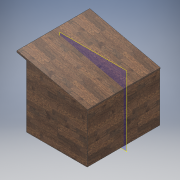
# Autodesk Inventor part: Top
Saved by Autodesk Inventor 2017 (Build 210142000, 142)
## iProperties
Created: 2016-09-09
Part Number: Top
Material: Generic
Document SubType Name: Modeling
Designer: s.ethan.wierenga
Density: 1 g/cm^3
Appearance: White Ash - Java
Author: s.ethan.wierenga
Autodesk Inventor part; units mm, degrees
ref_plane "YZ Plane" through (0, 0, 0) normal (1, 0, 0) x (0, 1, 0)
ref_plane "XZ Plane" through (0, 0, 0) normal (0, 1, 0) x (-1, 0, 0)
ref_plane "XY Plane" through (0, 0, 0) normal (0, 0, 1) x (1, 0, 0)
sketch "Sketch1" plane through (0, 0, 0) normal (0, 1, 0) x (-1, 0, 0)
  line L0 (0, 0) -> (-762, 0)
  line L1 (-762, 0) -> (-762, -914.4)
  line L2 (-762, -914.4) -> (0, -914.4)
  line L3 (0, -914.4) -> (0, 0)
  dimension "d0" = 762
  dimension "d1" = 914.4
  constraints: 8 end point, 2 parallel, 1 horizontal, 1 perpendicular
  measures "d0" distance of L2.end L1.end
  measures "d1" distance of L1.end L0.end
extrude "Extrusion1" add sketch "Sketch1" along normal blind 19.05
sketch "Sketch5" plane through (762, 0, -914.4) normal (0, 0, -1) x (-1, 0, 0)
  line L0 (0, 0) -> (0, 19.05) projected
  line L1 (0, 0) -> (762, 0) projected
  line L2 (762, 0) -> (762, 19.05) projected
  line L3 (762, 628.65) -> (762, 781.05)
  line L4 (762, 781.05) -> (0, 609.6)
  line L5 (0, 609.6) -> (762, 609.6) construction
  line L6 (762, 19.05) -> (762, 628.65) construction
  line L7 (762, 781.05) -> (757.8183, 799.6354)
  line L8 (757.8183, 799.6354) -> (-4.1817, 628.1854)
  line L9 (0, 609.6) -> (84.6693, 628.65) projected
  line L10 (-4.1817, 628.1854) -> (0, 609.6)
  line L11 (0, 19.05) -> (762, 19.05) projected
  dimension "d22" = 152.4
  dimension "d23" = 12.68
  dimension "d25" = 19.05
  dimension "d26" = 90
  dimension "d28" = 90
  dimension "d29" = 90
  constraints: 12 end point, 1 perpendicular, 1 point on line, 1 vertical
  measures "d22" distance of L3.start L3.end
  measures "d23" angle of L5 L4
  measures "d25" distance of L3.end L7.end
  measures "d26" angle of L7 L4
  measures "d28" angle of L4 L10
  measures "d29" angle of L8 L10
extrude "Extrusion5" add sketch "Sketch5" against normal up to surface (914.4 mm away) contours L4 L10 L8 L7
sketch "Sketch7" plane through (0, 19.05, 0) normal (0, 1, 0) x (1, 0, 0)
  line L0 (0, 0) -> (762, 0) projected
  line L1 (0, 914.4) -> (0, 0) projected
  line L2 (762, 914.4) -> (0, 914.4) projected
  line L3 (762, 0) -> (762, 914.4) projected
  line L4 (762, 0) -> (762, 914.4) projected
  line L5 (0, 914.4) -> (0, 0) projected
  line L6 (762, 914.4) -> (0, 914.4)
  line L7 (0, 914.4) -> (0, 895.35)
  line L8 (0, 895.35) -> (742.95, 895.35)
  line L9 (762, 895.35) -> (762, 914.4)
  line L10 (762, 914.4) -> (742.95, 914.4)
  line L11 (742.95, 895.35) -> (742.95, 457.2)
  line L12 (742.95, 457.2) -> (762, 457.2)
  line L13 (762, 457.2) -> (762, 914.4)
  dimension "d38" = 19.05
  dimension "d39" = 19.05
  dimension "d40" = 457.2
  constraints: 16 end point, 4 parallel, 2 horizontal, 2 perpendicular, 1 point on line
  measures "d38" distance of L7.end L6.end
  measures "d39" distance of L12.end L11.end
  measures "d40" distance of L11.end L10.end
extrude "Extrusion7" add sketch "Sketch7" along normal blind 609.6 contours L1 L2 L3 L12 L11 L8
sketch "Sketch8" plane through (762, 0, -914.4) normal (0, 0, -1) x (-1, 0, 0)
  line L0 (0, 0) -> (762, 0) projected
  line L1 (762, 0) -> (762, 628.65) projected
  line L2 (84.6667, 628.65) -> (762, 628.65) projected
  line L3 (84.6667, 628.65) -> (762, 781.05) projected
  line L4 (762, 781.05) -> (757.8183, 799.6354) projected
  line L5 (757.8183, 799.6354) -> (-4.1817, 628.1854) projected
  line L6 (-4.1817, 628.1854) -> (0, 609.6) projected
  line L7 (0, 0) -> (0, 609.6) projected
  line L8 (762, 628.65) -> (762, 781.05)
  line L9 (84.6667, 628.65) -> (762, 781.05) projected
  line L10 (762, 781.05) -> (84.6667, 628.65)
  line L11 (84.6667, 628.65) -> (762, 628.65)
  constraints: 6 end point, 1 collinear, 1 perpendicular, 1 vertical
extrude "Extrusion8" add sketch "Sketch8" against normal blind 19.05 contours L2 L3 L8
ref_plane "Work Plane2" through (762, 0, -457.2) normal (0, 0, -1) x (-1, 0, 0)
mirror "Mirror1" about plane through (762, 0, -457.2) normal (0, 0, -1) of "Extrusion7"
sketch "Sketch9" plane through (0, 0, 0) normal (0, 0, 1) x (1, 0, 0)
  line L0 (766.1817, 628.1854) -> (762, 609.6) projected
  line L1 (4.1817, 799.6354) -> (766.1817, 628.1854) projected
  line L2 (0, 781.05) -> (4.1817, 799.6354) projected
  line L3 (677.3333, 628.65) -> (0, 781.05) projected
  line L4 (677.3333, 628.65) -> (0, 628.65) projected
  line L5 (0, 0) -> (0, 628.65) projected
  line L6 (0, 0) -> (762, 0) projected
  line L7 (762, 0) -> (762, 609.6) projected
  line L8 (0, 19.05) -> (0, 781.05) projected
  line L9 (0, 628.65) -> (0, 781.05)
  line L10 (0, 781.05) -> (677.3333, 628.65)
  line L11 (0, 781.05) -> (742.95, 613.8863) projected
  line L12 (0, 628.65) -> (677.3333, 628.65)
  constraints: 6 end point, 2 collinear, 1 perpendicular
extrude "Extrusion9" add sketch "Sketch9" against normal blind 19.05 contours L3 L4 L8
sketch "Sketch12" plane through (742.95, 19.05, -895.35) normal (-1, 0, 0) x (0, 0, 1)
  line L0 (0, 594.8363) -> (876.3, 594.8363) projected
  line L1 (0, 0) -> (0, 594.8363) projected
  line L2 (876.3, 0) -> (0, 0) projected
  line L3 (876.3, 0) -> (876.3, 594.8363) projected
  line L4 (0, 0) -> (0, 594.8363) projected
  line L5 (876.3, 0) -> (876.3, 762) projected
  line L6 (0, 442.4363) -> (876.3, 442.4363)
  line L7 (876.3, 442.4363) -> (876.3, 423.3862)
  line L8 (876.3, 423.3862) -> (0, 423.3862)
  line L9 (0, 423.3862) -> (0, 442.4363)
  point P0 (895.35, -19.05)
  dimension "d57" = 19.05
  dimension "d58" = 152.4
  constraints: 8 end point, 2 parallel, 2 point on line, 1 horizontal, 1 perpendicular
  measures "d57" distance of L6.end L7.end
  measures "d58" distance between parallel lines of L0 L6
extrude "Extrusion10" add sketch "Sketch12" along normal up to surface (742.95 mm away) contours L6 L3 L8 L1
sketch "Sketch13" plane through (742.95, 461.4863, -19.05) normal (0, 1, 0) x (1, 0, 0)
  line L0 (-742.95, 0) -> (-742.95, 876.3) projected
  line L1 (0, 876.3) -> (-742.95, 876.3) projected
  line L2 (0, 0) -> (0, 876.3) projected
  line L3 (-742.95, 0) -> (0, 0) projected
  line L4 (0, 0) -> (0, 876.3) projected
  line L5 (-742.95, 876.3) -> (-742.95, 0) projected
  line L6 (0, 438.15) -> (-742.95, 438.15)
  line L7 (-742.95, 438.15) -> (-742.95, 419.1)
  line L8 (-742.95, 419.1) -> (0, 419.1)
  line L9 (0, 419.1) -> (0, 438.15)
  point P0 (-742.95, -19.05)
  dimension "d61" = 19.05
  constraints: 8 end point, 2 parallel, 1 horizontal, 1 midpoint, 1 perpendicular, 1 point on line
  measures "d61" distance of L7.end L6.end
extrude "Extrusion11" add sketch "Sketch13" along normal up to surface contours L0 L6 L2 L8 surface through (0, 781.05, -914.4) normal (-0.2195, -0.9756, 0)
sketch "Sketch14" plane through (4.1817, 799.6354, -914.4) normal (-0.9756, 0.2195, 0) x (0, 0, 1)
  line L0 (914.4, -19.05) -> (914.4, 0) projected
  line L1 (0, 0) -> (914.4, 0) projected
  line L2 (0, -19.05) -> (0, 0) projected
  line L3 (0, -19.05) -> (19.05, -19.05) projected
  line L4 (19.05, -19.05) -> (457.2, -19.05) projected
  line L5 (457.2, -19.05) -> (476.25, -19.05) projected
  line L6 (476.25, -19.05) -> (895.35, -19.05) projected
  line L7 (895.35, -19.05) -> (914.4, -19.05) projected
  line L8 (914.4, -781.05) -> (914.4, -19.05) projected
  line L9 (0, 0) -> (914.4, 0)
  line L10 (914.4, 0) -> (914.4, -19.05)
  line L11 (914.4, -19.05) -> (0, -19.05)
  line L12 (0, -19.05) -> (0, 0)
  constraints: 8 end point, 2 parallel, 1 horizontal, 1 perpendicular
extrude "Extrusion12" add sketch "Sketch14" along normal blind 127
sketch "Sketch15" plane through (742.95, 19.05, -895.35) normal (-1, 0, 0) x (0, 0, 1)
  line L0 (876.3, 423.3862) -> (0, 423.3862) projected
  line L1 (0, 0) -> (0, 423.3862) projected
  line L2 (876.3, 0) -> (0, 0) projected
  line L3 (876.3, 0) -> (876.3, 423.3862) projected
  line L4 (876.3, 423.3862) -> (0, 423.3862) projected
  line L5 (0, 0) -> (876.3, 0) projected
  line L6 (438.15, 423.3862) -> (457.2, 423.3862)
  line L7 (457.2, 423.3862) -> (457.2, 0)
  line L8 (457.2, 0) -> (438.15, 0)
  line L9 (438.15, 0) -> (438.15, 423.3862)
  point P0 (895.35, -19.05)
  dimension "d66" = 19.05
  constraints: 8 end point, 2 parallel, 1 horizontal, 1 midpoint, 1 perpendicular, 1 point on line
  measures "d66" distance of L7.end L8.end
extrude "Extrusion13" add sketch "Sketch15" along normal up to surface (742.95 mm away) contours L7 L2 L9 L0
sketch "Sketch16" plane through (742.95, 19.05, -438.15) normal (0, 0, 1) x (1, 0, 0)
  line L0 (-742.95, 0) -> (-742.95, 423.3862) projected
  line L1 (0, 423.3862) -> (-742.95, 423.3862) projected
  line L2 (0, 0) -> (0, 423.3862) projected
  line L3 (-742.95, 0) -> (0, 0) projected
  line L4 (0, 0) -> (0, 423.3862) projected
  line L5 (-742.95, 277.3362) -> (0, 277.3362)
  line L6 (0, 277.3362) -> (0, 296.3862)
  line L7 (0, 296.3862) -> (-742.95, 296.3862)
  line L8 (-742.95, 296.3862) -> (-742.95, 277.3362)
  line L9 (-742.95, 150.3362) -> (0, 150.3362)
  line L10 (0, 150.3362) -> (0, 131.2862)
  line L11 (0, 131.2862) -> (-742.95, 131.2862)
  line L12 (-742.95, 131.2862) -> (-742.95, 150.3362)
  point P0 (-742.95, -19.05)
  dimension "d69" = 19.05
  dimension "d70" = 127
  dimension "d71" = 19.05
  dimension "d72" = 127
  constraints: 16 end point, 4 parallel, 4 point on line, 2 horizontal, 2 perpendicular
  measures "d69" distance of L6.end L5.end
  measures "d70" distance between parallel lines of L1 L7
  measures "d71" distance of L9.end L10.end
  measures "d72" distance between parallel lines of L5 L9
extrude "Extrusion14" add sketch "Sketch16" along normal up to surface (419.1 mm away) contours L0 L9 L2 L11 | L0 L7 L2 L5
sketch "Sketch17" plane through (742.95, 19.05, -457.2) normal (0, 0, -1) x (-1, 0, 0)
  line L0 (742.95, 423.3862) -> (0, 423.3862) projected
  line L1 (0, 0) -> (742.95, 0) projected
  line L2 (0, 131.2862) -> (0, 0) projected
  line L3 (0, 277.3362) -> (0, 150.3362) projected
  line L4 (0, 423.3862) -> (0, 296.3862) projected
  line L5 (742.95, 423.3862) -> (742.95, 296.3862) projected
  line L6 (742.95, 277.3362) -> (742.95, 150.3362) projected
  line L7 (742.95, 131.2862) -> (742.95, 0) projected
  line L8 (0, 423.3862) -> (742.95, 0) construction
  line L9 (742.95, 423.3862) -> (0, 0) construction
  line L10 (0, 202.1681) -> (742.95, 202.1681)
  line L11 (742.95, 202.1681) -> (742.95, 221.2181)
  line L12 (742.95, 221.2181) -> (0, 221.2181)
  line L13 (0, 221.2181) -> (0, 202.1681)
  line L14 (0, 202.1681) -> (742.95, 221.2181) construction
  line L15 (742.95, 202.1681) -> (0, 221.2181) construction
  point P0 (742.95, -19.05)
  point P1 (371.475, 211.6931)
  dimension "d75" = 19.05
  constraints: 16 end point, 3 midpoint, 2 parallel, 1 horizontal, 1 perpendicular, 1 point on line
  measures "d75" distance of L11.end L10.end
extrude "Extrusion15" add sketch "Sketch17" along normal up to surface (438.15 mm away)
sketch "Sketch18" plane through (0, 0, -914.4) normal (-1, 0, 0) x (0, 0, 1)
  line L0 (476.25, 442.4362) -> (476.25, 315.4362) projected
  line L1 (19.05, 240.2681) -> (19.05, 442.4362) projected
  line L2 (457.2, 442.4362) -> (19.05, 442.4362) projected
  line L3 (457.2, 240.2681) -> (457.2, 442.4362) projected
  line L4 (457.2, 240.2681) -> (19.05, 240.2681) projected
  line L5 (476.25, 296.3862) -> (476.25, 169.3862) projected
  line L6 (476.25, 296.3862) -> (895.35, 296.3862) projected
  line L7 (895.35, 169.3862) -> (895.35, 296.3862) projected
  line L8 (476.25, 169.3862) -> (895.35, 169.3862) projected
  line L9 (476.25, 150.3362) -> (895.35, 150.3362) projected
  line L10 (895.35, 19.05) -> (895.35, 150.3362) projected
  line L11 (476.25, 19.05) -> (895.35, 19.05) projected
  line L12 (476.25, 150.3362) -> (476.25, 19.05) projected
  line L13 (476.25, 315.4362) -> (895.35, 315.4362) projected
  line L14 (476.25, 442.4362) -> (476.25, 315.4362) projected
  line L15 (895.35, 442.4362) -> (476.25, 442.4362) projected
  line L16 (895.35, 315.4362) -> (895.35, 442.4362) projected
  line L17 (19.05, 461.4863) -> (19.05, 781.05) projected
  line L18 (0, 781.05) -> (19.05, 781.05) projected
  line L19 (0, 0) -> (0, 781.05) projected
  line L20 (0, 0) -> (914.4, 0) projected
  line L21 (914.4, 0) -> (914.4, 781.05) projected
  line L22 (895.35, 781.05) -> (914.4, 781.05) projected
  line L23 (895.35, 461.4863) -> (895.35, 781.05) projected
  line L24 (476.25, 461.4863) -> (895.35, 461.4863) projected
  line L25 (476.25, 461.4863) -> (476.25, 781.05) projected
  line L26 (457.2, 781.05) -> (476.25, 781.05) projected
  line L27 (457.2, 461.4863) -> (457.2, 781.05) projected
  line L28 (19.05, 461.4863) -> (457.2, 461.4863) projected
  line L29 (457.2, 221.2181) -> (19.05, 221.2181) projected
  line L30 (457.2, 19.05) -> (457.2, 221.2181) projected
  line L31 (19.05, 19.05) -> (457.2, 19.05) projected
  line L32 (19.05, 19.05) -> (19.05, 221.2181) projected
  line L33 (19.05, 461.4863) -> (19.05, 613.8863) projected
  line L34 (457.2, 240.2681) -> (457.2, 442.4362) projected
  line L35 (19.05, 461.4863) -> (457.2, 461.4863)
  line L36 (457.2, 461.4863) -> (457.2, 442.4362)
  line L37 (457.2, 442.4362) -> (19.05, 442.4362)
  line L38 (19.05, 442.4362) -> (19.05, 461.4863)
  line L39 (457.2, 240.2681) -> (19.05, 240.2681) projected
  line L40 (457.2, 221.2181) -> (19.05, 221.2181) projected
  line L41 (19.05, 240.2681) -> (457.2, 240.2681)
  line L42 (457.2, 240.2681) -> (457.2, 221.2181)
  line L43 (457.2, 221.2181) -> (19.05, 221.2181)
  line L44 (19.05, 221.2181) -> (19.05, 240.2681)
  line L45 (476.25, 461.4863) -> (476.25, 781.05) projected
  line L46 (895.35, 315.4362) -> (895.35, 442.4362) projected
  line L47 (476.25, 461.4863) -> (895.35, 461.4863)
  line L48 (895.35, 461.4863) -> (895.35, 442.4362)
  line L49 (895.35, 442.4362) -> (476.25, 442.4362)
  line L50 (476.25, 442.4362) -> (476.25, 461.4863)
  line L51 (895.35, 169.3862) -> (895.35, 296.3862) projected
  line L52 (476.25, 315.4362) -> (895.35, 315.4362)
  line L53 (895.35, 315.4362) -> (895.35, 296.3862)
  line L54 (895.35, 296.3862) -> (476.25, 296.3862)
  line L55 (476.25, 296.3862) -> (476.25, 315.4362)
  line L56 (476.25, 169.3862) -> (895.35, 169.3862) projected
  line L57 (895.35, 19.05) -> (895.35, 150.3362) projected
  line L58 (476.25, 169.3862) -> (895.35, 169.3862)
  line L59 (895.35, 169.3862) -> (895.35, 150.3362)
  line L60 (895.35, 150.3362) -> (476.25, 150.3362)
  line L61 (476.25, 150.3362) -> (476.25, 169.3862)
  constraints: 40 end point, 10 parallel, 5 horizontal, 5 perpendicular
extrude "Extrusion16" cut sketch "Sketch18" against normal blind 12.7 contours L50 L24 L48 L15 | L13 L53 L6 L55 | L8 L59 L9 L61 | L36 L2 L38 L28 | L42 L29 L44 L4
body "Solid1"
